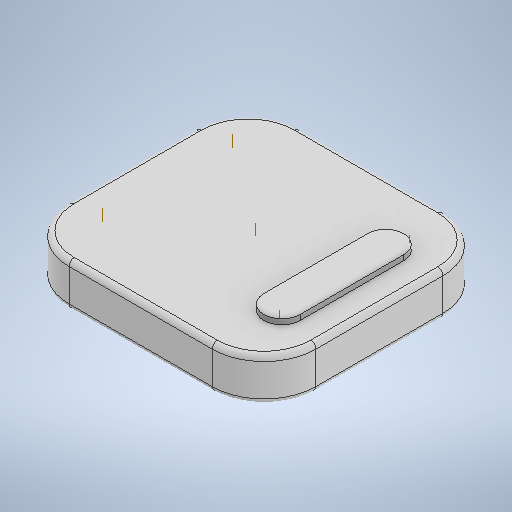
# Autodesk Inventor part: Pin-Low-Fidelity
Saved by Autodesk Inventor 2025 (Build 290162000, 162)
## iProperties
Created: 2025-03-04
Part Number: Pin-Low-Fidelity
Material: Generic
Document SubType Name: Modeling
Designer: maxsm
Density: 1 g/cm^3
Appearance: Default
Author: maxsm
Autodesk Inventor part; units mm, degrees
ref_plane "YZ Plane" through (0, 0, 0) normal (1, 0, 0) x (0, 1, 0)
ref_plane "XZ Plane" through (0, 0, 0) normal (0, 1, 0) x (-1, 0, 0)
ref_plane "XY Plane" through (0, 0, 0) normal (0, 0, 1) x (1, 0, 0)
sketch "Sketch1" plane through (0, 0, 0) normal (0, 1, 0) x (-1, 0, 0)
  line L0 (13.8, 22.25) -> (-13.8, 22.25)
  line L1 (-23.8, 12.25) -> (-23.8, -12.25)
  line L2 (-13.8, -22.25) -> (13.8, -22.25)
  line L3 (23.8, -12.25) -> (23.8, 12.25)
  line L4 (23.8, 22.25) -> (-23.8, -22.25) construction
  line L5 (-23.8, 22.25) -> (23.8, -22.25) construction
  arc A0 (23.8, 12.25) -> (13.8, 22.25) centre (13.8, 12.25) ccw
  arc A1 (13.8, -22.25) -> (23.8, -12.25) centre (13.8, -12.25) ccw
  arc A2 (-23.8, -12.25) -> (-13.8, -22.25) centre (-13.8, -12.25) ccw
  arc A3 (-13.8, 22.25) -> (-23.8, 12.25) centre (-13.8, 12.25) ccw
  point P0 (0, 0)
  dimension "d0" = 47.6
  dimension "d1" = 44.5
  dimension "d3" = 10
  constraints: 12 end point, 8 point on circle, 8 point on line, 8 tangent, 4 centre point, 3 equal radius, 2 midpoint, 2 parallel, 1 horizontal, 1 perpendicular
  measures "d0" distance of L5.end L4.end
  measures "d1" distance of L4.end L5.start
  measures "d3" distance from line of L3.end L0
extrude "Extrusion1" add sketch "Sketch1" along normal blind 8.25
fillet "Fillet1" radius 1 16 edges at (20.8711, 0, 19.3211) (23.8, 0, 0) (20.8711, 0, -19.3211) (0, 0, -22.25) (-20.8711, 0, -19.3211) (-23.8, 0, 0) (-20.8711, 0, 19.3211) (0, 0, 22.25) (23.8, 8.25, 0) (20.8711, 8.25, -19.3211) (0, 8.25, -22.25) (-20.8711, 8.25, -19.3211) (-23.8, 8.25, 0) (-20.8711, 8.25, 19.3211) (0, 8.25, 22.25) (20.8711, 8.25, 19.3211)
sketch "Sketch2" plane through (0, 0, 0) normal (0, -1, 0) x (1, 0, 0)
  line L0 (-33.32, 0) -> (33.32, 0) projected
  line L1 (0, -31.15) -> (0, 31.15) projected
  point P0 (0, 0)
  point P1 (17, 12.5)
  point P2 (17, -12.5)
  point P3 (-17, 12.5)
  point P4 (-17, -12.5)
  dimension "d7" = 25
  dimension "d8" = 34
  constraints: 2 symmetric about line, 1 horizontal alignment, 1 vertical alignment
  measures "d7" distance of point (17, -12.5) point (17, 12.5)
  measures "d8" distance of point (-17, 12.5) point (17, 12.5)
sketch "Sketch3" plane through (0, 0, 0) normal (0, -1, 0) x (1, 0, 0)
  line L0 (1.3258, -1.3258) -> (-1.3258, 1.3258) construction
  line L1 (1.7678, -0.8839) -> (-0.8839, 1.7678)
  line L2 (-1.7678, 0.8839) -> (0.8839, -1.7678)
  arc A0 (0.8839, -1.7678) -> (1.7678, -0.8839) centre (1.3258, -1.3258) ccw
  arc A1 (-0.8839, 1.7678) -> (-1.7678, 0.8839) centre (-1.3258, 1.3258) ccw
  line L3 (0, -31.15) -> (0, 31.15) projected
  point P0 (0, 0)
  point P1 (-1.7678, 1.7678)
  point P2 (1.7678, -1.7678)
  dimension "d9" = 5
  dimension "d10" = 1.25
  dimension "d11" = 135
  constraints: 8 end point, 6 point on circle, 4 tangent, 2 centre point, 1 midpoint, 1 parallel
  measures "d9" distance of point (-1.768, 1.768) point (1.768, -1.768)
  measures "d10" distance between parallel lines of L2 L1
  measures "d11" angle of L1 L3
extrude "Extrusion2" cut sketch "Sketch3" against normal blind 0.5
sketch "Sketch5" plane through (0, 8.25, 0) normal (0, 1, 0) x (1, 0, 0)
  line L0 (15, 10) -> (15, -10) construction
  line L1 (11.5, 10) -> (11.5, -10)
  line L2 (18.5, -10) -> (18.5, 10)
  arc A0 (18.5, 10) -> (11.5, 10) centre (15, 10) ccw
  arc A1 (11.5, -10) -> (18.5, -10) centre (15, -10) ccw
  point P0 (0, 0)
  point P1 (15, 0)
  dimension "d16" = 10
  dimension "d17" = 7
  dimension "d18" = 15
  constraints: 8 end point, 4 point on circle, 4 tangent, 2 centre point, 1 horizontal alignment, 1 midpoint, 1 parallel, 1 vertical
  measures "d16" distance of point (15, 0) L0.end
  measures "d17" diameter of A1
  measures "d18" distance of point (0, 0) point (15, 0)
extrude "Extrusion4" add sketch "Sketch5" along normal blind 1
body "Solid1"
